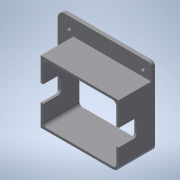
# Autodesk Inventor part: SP49V1 Protector Pasador
Saved by Autodesk Inventor 2021.2 (Build 252289000, 289)
## iProperties
Created: 2026-09-07
Part Number: SP49V1 Protector Pasador
Material: Generic
Document SubType Name: Modeling
Designer: nelso
Density: 1 g/cm^3
Appearance: Default
Author: nelso
Autodesk Inventor part; units mm, degrees
ref_plane "YZ Plane" through (0, 0, 0) normal (1, 0, 0) x (0, 1, 0)
ref_plane "XZ Plane" through (0, 0, 0) normal (0, 1, 0) x (-1, 0, 0)
ref_plane "XY Plane" through (0, 0, 0) normal (0, 0, 1) x (1, 0, 0)
sketch "Sketch1" plane through (0, 0, 0) normal (0, 1, 0) x (-1, 0, 0)
  line L0 (32.35, 26) -> (-32.35, 26)
  line L1 (-32.35, 26) -> (-32.35, -26)
  line L2 (-32.35, -26) -> (32.35, -26)
  line L3 (32.35, -26) -> (32.35, 26)
  line L4 (32.35, 26) -> (-32.35, -26) construction
  line L5 (-32.35, 26) -> (32.35, -26) construction
  point P0 (0, 0)
  dimension "d0" = 64.7
  dimension "d1" = 52
  constraints: 12 end point, 2 midpoint, 2 parallel, 1 horizontal, 1 perpendicular
  measures "d0" distance of L2.end L1.end
  measures "d1" distance of L1.end L0.end
extrude "Extrusion1" add sketch "Sketch1" along normal mid plane 30
shell "Shell1" thickness 2 removed faces 2 at (10.7833, 15, 8.6667) at (10.7833, -15, 8.6667)
sketch "Sketch3" plane through (32.35, -15, 26) normal (1, 0, 0) x (0, 0, -1)
  line L0 (0, 30) -> (0, 0) projected
  line L1 (0, 0) -> (19.9, 0)
  line L2 (2, 0) -> (50, 0) projected
  line L3 (19.9, 0) -> (33.9, 0)
  line L4 (33.9, 0) -> (33.9, 15)
  line L5 (33.9, 15) -> (19.9, 15)
  line L6 (19.9, 15) -> (19.9, 0)
  point P0 (26, 15)
  point P1 (0, 27)
  point P2 (33.9, 0)
  dimension "d12" = 19.9
  dimension "d13" = 14
  dimension "d14" = 15
  constraints: 10 end point, 2 parallel, 1 horizontal, 1 perpendicular, 1 point on line
  measures "d12" distance of L0.end L1.end
  measures "d13" distance of L5.end L4.end
  measures "d14" distance of L4.end L3.end
extrude "Extrusion3" cut sketch "Sketch3" against normal through all
sketch "Sketch4" plane through (0, 15, 0) normal (0, 1, 0) x (1, 0, 0)
  line L0 (32.35, -26) -> (32.35, 26) projected
  line L1 (30.35, -24) -> (-30.35, -24) projected
  line L2 (32.35, 26) -> (-30.35, 26)
  line L3 (-30.35, 26) -> (-30.35, -24)
  line L4 (-30.35, -24) -> (32.35, -24)
  line L5 (32.35, -24) -> (32.35, 26)
  line L6 (32.35, 26) -> (-32.35, 26) projected
  line L7 (32.35, 26) -> (-45.35, 26)
  line L8 (-45.35, 26) -> (-45.35, -39)
  line L9 (-45.35, -39) -> (32.35, -39)
  line L10 (32.35, -39) -> (32.35, 26)
  point P0 (0, 0)
  dimension "d17" = 77.7
  dimension "d18" = 65
  constraints: 16 end point, 4 parallel, 2 horizontal, 2 perpendicular
  measures "d17" distance of L9.end L8.end
  measures "d18" distance of L8.end L7.end
extrude "Extrusion4" add sketch "Sketch4" against normal blind 3 contours L10 L9 L8 L7 L6 L3 L1 L4 L0
fillet "Fillet1" radius 3 10 edges at (-30.35, 0, 24) (-30.35, 0, -24) (-31.35, 0, -7.9) (-31.35, 0, 6.1) (31.35, 0, -7.9) (31.35, 0, 6.1) (30.35, 0, -24) (30.35, 0, 24) (32.35, 13.5, 39) (-45.35, 13.5, -26)
fillet "Fillet1" radius 6 1 edges at (-45.35, 13.5, 39)
fillet "Fillet1" radius 4.5 1 edges at (32.35, 0, -26)
sketch "Sketch5" plane through (0, 15, 0) normal (0, 1, 0) x (1, 0, 0)
  line L0 (-30.35, -21) -> (-30.35, 21) projected
  line L1 (-45.35, 26) -> (-30.35, 26)
  line L2 (-30.35, 26) -> (-30.35, 11)
  line L3 (-30.35, 11) -> (-45.35, 11)
  line L4 (-45.35, 11) -> (-45.35, 26)
  arc A0 (-30.35, -21) -> (-27.35, -24) centre (-27.35, -21) ccw projected
  line L5 (-45.35, -39) -> (-27.35, -39)
  line L6 (-27.35, -39) -> (-27.35, -21)
  line L7 (-27.35, -21) -> (-45.35, -21)
  line L8 (-45.35, -21) -> (-45.35, -39)
  line L9 (27.35, -24) -> (-27.35, -24) projected
  line L10 (32.35, -39) -> (17.35, -39)
  line L11 (17.35, -39) -> (17.35, -24)
  line L12 (17.35, -24) -> (32.35, -24)
  line L13 (32.35, -24) -> (32.35, -39)
  point P0 (0, 0)
  point P1 (-37.85, 18.5)
  point P2 (-36.35, -30)
  point P3 (24.85, -31.5)
  dimension "d23" = 15
  dimension "d24" = 15
  constraints: 24 end point, 6 parallel, 4 point on line, 3 horizontal, 3 perpendicular
  measures "d23" distance of L1.end L2.end
  measures "d24" distance of L11.end L12.end
hole "Hole1" at (-37.85, 15, -18.5) at (-36.35, 15, 30) at (24.85, 15, 31.5) direction (0, -1, 0) diameter 3.6 depth 8 tip angle 118 clearance for "Countersunk Flat Head Screw ISO 2009/7046" size "M3" standard "ISO"
sketch "Sketch6" plane through (0, 15, 0) normal (0, 1, 0) x (1, 0, 0)
  line L0 (-17.647, -28.2352) -> (10.9204, -28.2352) construction
  line L1 (10.9204, -28.2352) -> (10.9204, -35.4601) construction
  line L2 (10.9204, -35.4601) -> (-17.647, -35.4601) construction
  line L3 (-17.647, -35.4601) -> (-17.647, -28.2352) construction
  line L4 (-14.9497, -31.809) -> (-17.284, -31.809)
  line L5 (-17.284, -31.809) -> (-17.284, -28.309)
  line L6 (-17.284, -28.309) -> (-16.4047, -28.309)
  line L7 (-16.4047, -28.309) -> (-16.4047, -31.1425)
  line L8 (-16.4047, -31.1425) -> (-14.9497, -31.1425)
  line L9 (-14.9497, -31.1425) -> (-14.9497, -31.809)
  spline S0 degree 2 poles (-11.3448, -30.059) (-11.3448, -30.9099) (-12.2524, -31.8827) (-13.0409, -31.8827) knots 0 0 0 1 2 2 2
  spline S1 degree 2 poles (-13.0409, -31.8827) (-13.8322, -31.8827) (-14.7341, -30.8985) (-14.7341, -30.059) knots 0 0 0 1 2 2 2
  spline S2 degree 2 poles (-14.7341, -30.059) (-14.7341, -29.2166) (-13.8322, -28.2352) (-13.0409, -28.2352) knots 0 0 0 1 2 2 2
  spline S3 degree 2 poles (-13.0409, -28.2352) (-12.2524, -28.2352) (-11.3448, -29.2109) (-11.3448, -30.059) knots 0 0 0 1 2 2 2
  spline S4 degree 2 poles (-12.2524, -30.059) (-12.2524, -29.7442) (-12.38, -29.3045) (-12.4906, -29.1655) knots 0 0 0 1 2 2 2
  spline S5 degree 2 poles (-12.4906, -29.1655) (-12.6012, -29.0209) (-12.8849, -28.8961) (-13.038, -28.8961) knots 0 0 0 1 2 2 2
  spline S6 degree 2 poles (-13.038, -28.8961) (-13.1997, -28.8961) (-13.4635, -29.0124) (-13.5854, -29.1599) knots 0 0 0 1 2 2 2
  spline S7 degree 2 poles (-13.5854, -29.1599) (-13.6932, -29.296) (-13.8265, -29.747) (-13.8265, -30.059) knots 0 0 0 1 2 2 2
  spline S8 degree 2 poles (-13.8265, -30.059) (-13.8265, -30.3823) (-13.6989, -30.8078) (-13.5883, -30.9524) knots 0 0 0 1 2 2 2
  spline S9 degree 2 poles (-13.5883, -30.9524) (-13.4777, -31.0971) (-13.1912, -31.2219) (-13.038, -31.2219) knots 0 0 0 1 2 2 2
  spline S10 degree 2 poles (-13.038, -31.2219) (-12.882, -31.2219) (-12.5927, -31.0886) (-12.4878, -30.9467) knots 0 0 0 1 2 2 2
  spline S11 degree 2 poles (-12.4878, -30.9467) (-12.3743, -30.7936) (-12.2524, -30.388) (-12.2524, -30.059) knots 0 0 0 1 2 2 2
  spline S12 degree 2 poles (-9.314, -31.8771) (-10.1025, -31.8771) (-11.0271, -30.9241) (-11.0271, -30.0618) knots 0 0 0 1 2 2 2
  spline S13 degree 2 poles (-11.0271, -30.0618) (-11.0271, -29.2308) (-10.0996, -28.2409) (-9.3111, -28.2409) knots 0 0 0 1 2 2 2
  spline S14 degree 2 poles (-9.3111, -28.2409) (-9.1041, -28.2409) (-8.7694, -28.2891) (-8.6162, -28.3288) knots 0 0 0 1 2 2 2
  spline S15 degree 2 poles (-8.6162, -28.3288) (-8.4971, -28.3657) (-8.2163, -28.4877) (-8.1284, -28.5331) knots 0 0 0 1 2 2 2
  line L10 (-8.1284, -28.5331) -> (-8.1284, -29.3669)
  line L11 (-8.1284, -29.3669) -> (-8.2163, -29.3669)
  spline S16 degree 2 poles (-8.2163, -29.3669) (-8.2815, -29.3102) (-8.4744, -29.1514) (-8.5964, -29.0776) knots 0 0 0 1 2 2 2
  spline S17 degree 2 poles (-8.5964, -29.0776) (-8.7183, -29.001) (-9.0105, -28.8961) (-9.1721, -28.8961) knots 0 0 0 1 2 2 2
  spline S18 degree 2 poles (-9.1721, -28.8961) (-9.3622, -28.8961) (-9.677, -29.0152) (-9.8217, -29.1655) knots 0 0 0 1 2 2 2
  spline S19 degree 2 poles (-9.8217, -29.1655) (-9.9521, -29.2989) (-10.1195, -29.7555) (-10.1195, -30.0647) knots 0 0 0 1 2 2 2
  spline S20 degree 2 poles (-10.1195, -30.0647) (-10.1195, -30.3908) (-9.9465, -30.8361) (-9.8046, -30.9723) knots 0 0 0 1 2 2 2
  spline S21 degree 2 poles (-9.8046, -30.9723) (-9.6685, -31.1056) (-9.3338, -31.2219) (-9.1665, -31.2219) knots 0 0 0 1 2 2 2
  spline S22 degree 2 poles (-9.1665, -31.2219) (-8.9935, -31.2219) (-8.6786, -31.1056) (-8.5708, -31.0347) knots 0 0 0 1 2 2 2
  spline S23 degree 2 poles (-8.5708, -31.0347) (-8.4517, -30.9638) (-8.273, -30.8134) (-8.2078, -30.7539) knots 0 0 0 1 2 2 2
  line L12 (-8.2078, -30.7539) -> (-8.1284, -30.7539)
  line L13 (-8.1284, -30.7539) -> (-8.1284, -31.5764)
  spline S24 degree 2 poles (-8.1284, -31.5764) (-8.2248, -31.6218) (-8.4773, -31.7352) (-8.6134, -31.7749) knots 0 0 0 1 2 2 2
  spline S25 degree 2 poles (-8.6134, -31.7749) (-8.7779, -31.826) (-9.0644, -31.8771) (-9.314, -31.8771) knots 0 0 0 1 2 2 2
  line L14 (-4.5433, -31.809) -> (-5.6069, -31.809)
  line L15 (-5.6069, -31.809) -> (-6.5571, -30.388)
  line L16 (-6.5571, -30.388) -> (-6.7301, -30.6262)
  line L17 (-6.7301, -30.6262) -> (-6.7301, -31.809)
  line L18 (-6.7301, -31.809) -> (-7.6093, -31.809)
  line L19 (-7.6093, -31.809) -> (-7.6093, -28.309)
  line L20 (-7.6093, -28.309) -> (-6.7301, -28.309)
  line L21 (-6.7301, -28.309) -> (-6.7301, -29.8718)
  line L22 (-6.7301, -29.8718) -> (-5.6069, -28.309)
  line L23 (-5.6069, -28.309) -> (-4.5944, -28.309)
  line L24 (-4.5944, -28.309) -> (-5.8423, -29.9342)
  line L25 (-5.8423, -29.9342) -> (-4.5433, -31.809)
  point P0 (0, 0)
  constraints: 2 other
extrude "Extrusion5" cut sketch "Sketch6" against normal blind 0.3
sketch "Sketch7" plane through (0, 15, 0) normal (0, 1, 0) x (1, 0, 0)
  line L0 (-27.35, 24) -> (27.35, 24) projected
  arc A0 (30.35, 21) -> (27.35, 24) centre (27.35, 21) ccw projected
  line L1 (30.35, 21) -> (30.35, -21) projected
  arc A1 (27.35, -24) -> (30.35, -21) centre (27.35, -21) ccw projected
  line L2 (27.35, -24) -> (-27.35, -24) projected
  arc A2 (-30.35, -21) -> (-27.35, -24) centre (-27.35, -21) ccw projected
  line L3 (-30.35, -21) -> (-30.35, 21) projected
  arc A3 (-27.35, 24) -> (-30.35, 21) centre (-27.35, 21) ccw projected
  arc A4 (32.35, 21.5) -> (27.85, 26) centre (27.85, 21.5) ccw projected
  line L4 (27.85, 26) -> (-42.35, 26) projected
  arc A5 (-42.35, 26) -> (-45.35, 23) centre (-42.35, 23) ccw projected
  line L5 (-45.35, 23) -> (-45.35, -33) projected
  arc A6 (-45.35, -33) -> (-39.35, -39) centre (-39.35, -33) ccw projected
  line L6 (-39.35, -39) -> (29.35, -39) projected
  arc A7 (29.35, -39) -> (32.35, -36) centre (29.35, -36) ccw projected
  line L7 (32.35, -36) -> (32.35, 21.5) projected
  circle A8 centre (24.85, -31.5) radius 1.8 projected
  circle A9 centre (-37.85, 18.5) radius 1.8 projected
  circle A10 centre (-36.35, -30) radius 1.8 projected
  line L8 (-5.8423, -29.9342) -> (-4.5433, -31.809) projected
  line L9 (-4.5433, -31.809) -> (-5.6069, -31.809) projected
  line L10 (-5.6069, -31.809) -> (-6.5571, -30.388) projected
  line L11 (-6.5571, -30.388) -> (-6.7301, -30.6262) projected
  line L12 (-6.7301, -30.6262) -> (-6.7301, -31.809) projected
  line L13 (-6.7301, -31.809) -> (-7.6093, -31.809) projected
  line L14 (-7.6093, -31.809) -> (-7.6093, -28.309) projected
  line L15 (-7.6093, -28.309) -> (-6.7301, -28.309) projected
  line L16 (-6.7301, -28.309) -> (-6.7301, -29.8718) projected
  line L17 (-6.7301, -29.8718) -> (-5.6069, -28.309) projected
  line L18 (-5.6069, -28.309) -> (-4.5944, -28.309) projected
  line L19 (-4.5944, -28.309) -> (-5.8423, -29.9342) projected
  line L20 (-14.9497, -31.1425) -> (-14.9497, -31.809) projected
  line L21 (-14.9497, -31.809) -> (-17.284, -31.809) projected
  line L22 (-17.284, -31.809) -> (-17.284, -28.309) projected
  line L23 (-17.284, -28.309) -> (-16.4047, -28.309) projected
  line L24 (-16.4047, -28.309) -> (-16.4047, -31.1425) projected
  line L25 (-16.4047, -31.1425) -> (-14.9497, -31.1425) projected
  spline S0 degree 2 poles (-13.0409, -28.2352) (-12.2524, -28.2352) (-11.3448, -29.2109) (-11.3448, -30.059) knots 0 0 0 0.5 1 1 1 projected
  spline S1 degree 2 poles (-11.3448, -30.059) (-11.3448, -30.9099) (-12.2524, -31.8827) (-13.0409, -31.8827) knots 0 0 0 0.5 1 1 1 projected
  spline S2 degree 2 poles (-13.0409, -31.8827) (-13.8322, -31.8827) (-14.7341, -30.8985) (-14.7341, -30.059) knots 0 0 0 0.5 1 1 1 projected
  spline S3 degree 2 poles (-14.7341, -30.059) (-14.7341, -29.2166) (-13.8322, -28.2352) (-13.0409, -28.2352) knots 0 0 0 0.5 1 1 1 projected
  spline S4 degree 2 poles (-8.6134, -31.7749) (-8.7779, -31.826) (-9.0644, -31.8771) (-9.314, -31.8771) knots 0 0 0 0.5 1 1 1 projected
  spline S5 degree 2 poles (-9.314, -31.8771) (-10.1025, -31.8771) (-11.0271, -30.9241) (-11.0271, -30.0618) knots 0 0 0 0.5 1 1 1 projected
  spline S6 degree 2 poles (-11.0271, -30.0618) (-11.0271, -29.2308) (-10.0996, -28.2409) (-9.3111, -28.2409) knots 0 0 0 0.5 1 1 1 projected
  spline S7 degree 2 poles (-9.3111, -28.2409) (-9.1041, -28.2409) (-8.7694, -28.2891) (-8.6162, -28.3288) knots 0 0 0 0.5 1 1 1 projected
  spline S8 degree 2 poles (-8.6162, -28.3288) (-8.4971, -28.3657) (-8.2163, -28.4877) (-8.1284, -28.5331) knots 0 0 0 0.5 1 1 1 projected
  line L26 (-8.1284, -28.5331) -> (-8.1284, -29.3669) projected
  line L27 (-8.1284, -29.3669) -> (-8.2163, -29.3669) projected
  spline S9 degree 2 poles (-8.2163, -29.3669) (-8.2815, -29.3102) (-8.4744, -29.1514) (-8.5964, -29.0776) knots 0 0 0 0.5 1 1 1 projected
  spline S10 degree 2 poles (-8.5964, -29.0776) (-8.7183, -29.001) (-9.0105, -28.8961) (-9.1721, -28.8961) knots 0 0 0 0.5 1 1 1 projected
  spline S11 degree 2 poles (-9.1721, -28.8961) (-9.3622, -28.8961) (-9.677, -29.0152) (-9.8217, -29.1655) knots 0 0 0 0.5 1 1 1 projected
  spline S12 degree 2 poles (-9.8217, -29.1655) (-9.9521, -29.2989) (-10.1195, -29.7555) (-10.1195, -30.0647) knots 0 0 0 0.5 1 1 1 projected
  spline S13 degree 2 poles (-10.1195, -30.0647) (-10.1195, -30.3908) (-9.9465, -30.8361) (-9.8046, -30.9723) knots 0 0 0 0.5 1 1 1 projected
  spline S14 degree 2 poles (-9.8046, -30.9723) (-9.6685, -31.1056) (-9.3338, -31.2219) (-9.1665, -31.2219) knots 0 0 0 0.5 1 1 1 projected
  spline S15 degree 2 poles (-9.1665, -31.2219) (-8.9935, -31.2219) (-8.6786, -31.1056) (-8.5708, -31.0347) knots 0 0 0 0.5 1 1 1 projected
  spline S16 degree 2 poles (-8.5708, -31.0347) (-8.4517, -30.9638) (-8.273, -30.8134) (-8.2078, -30.7539) knots 0 0 0 0.5 1 1 1 projected
  line L28 (-8.2078, -30.7539) -> (-8.1284, -30.7539) projected
  line L29 (-8.1284, -30.7539) -> (-8.1284, -31.5764) projected
  spline S17 degree 2 poles (-8.1284, -31.5764) (-8.2248, -31.6218) (-8.4773, -31.7352) (-8.6134, -31.7749) knots 0 0 0 0.5 1 1 1 projected
  spline S18 degree 2 poles (-12.4906, -29.1655) (-12.6012, -29.0209) (-12.8849, -28.8961) (-13.038, -28.8961) knots 0 0 0 0.5 1 1 1 projected
  spline S19 degree 2 poles (-13.038, -28.8961) (-13.1997, -28.8961) (-13.4635, -29.0124) (-13.5854, -29.1599) knots 0 0 0 0.5 1 1 1 projected
  spline S20 degree 2 poles (-13.5854, -29.1599) (-13.6932, -29.296) (-13.8265, -29.747) (-13.8265, -30.059) knots 0 0 0 0.5 1 1 1 projected
  spline S21 degree 2 poles (-13.8265, -30.059) (-13.8265, -30.3823) (-13.6989, -30.8078) (-13.5883, -30.9524) knots 0 0 0 0.5 1 1 1 projected
  spline S22 degree 2 poles (-13.5883, -30.9524) (-13.4777, -31.0971) (-13.1912, -31.2219) (-13.038, -31.2219) knots 0 0 0 0.5 1 1 1 projected
  spline S23 degree 2 poles (-13.038, -31.2219) (-12.882, -31.2219) (-12.5927, -31.0886) (-12.4878, -30.9467) knots 0 0 0 0.5 1 1 1 projected
  spline S24 degree 2 poles (-12.4878, -30.9467) (-12.3743, -30.7936) (-12.2524, -30.388) (-12.2524, -30.059) knots 0 0 0 0.5 1 1 1 projected
  spline S25 degree 2 poles (-12.2524, -30.059) (-12.2524, -29.7442) (-12.38, -29.3045) (-12.4906, -29.1655) knots 0 0 0 0.5 1 1 1 projected
  point P0 (0, 0)
  constraints: 26 other
extrude "Extrusion6" add sketch "Sketch7" against normal blind 0.3 separate body contours L8 L9 L10 L11 L12 L13 L14 L15 L16 L17 L18 L19 | L20 L21 L22 L23 L24 L25 | S0 S1 S2 S3 | S4 S5 S6 S7 S8 L26 L27 S9 S10 S11 S12 S13 S14 S15 S16 L28 L29 S17
body "Solid1"
body "Solid2"
